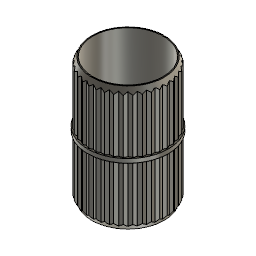
complete-v2-connector-pipe (Autodesk Fusion 360 design; units mm, degrees)
Autodesk Fusion 360 part; units mm, degrees
ref_plane "Arbeitsebene1" through (0, 0, -30) normal (0, 0, 1) x (1, 0, 0)
sketch "Skizze1" plane through (0, 0, -30) normal (0, 0, 1) x (1, 0, 0)
  circle A0 centre (0, 0) radius 17
  line L0 (19, 0) -> (18.33, 1.6037)
  line L1 (18.33, 1.6037) -> (18.7113, 3.2993)
  line L2 (18.7113, 3.2993) -> (17.773, 4.7623)
  line L3 (17.773, 4.7623) -> (17.8542, 6.4984)
  line L4 (17.8542, 6.4984) -> (16.6761, 7.7762)
  line L5 (16.6761, 7.7762) -> (16.4545, 9.5)
  line L6 (16.4545, 9.5) -> (15.0724, 10.5538)
  line L7 (15.0724, 10.5538) -> (14.5548, 12.213)
  line L8 (14.5548, 12.213) -> (13.0108, 13.0108)
  line L9 (13.0108, 13.0108) -> (12.213, 14.5548)
  line L10 (12.213, 14.5548) -> (10.5538, 15.0724)
  line L11 (10.5538, 15.0724) -> (9.5, 16.4545)
  line L12 (9.5, 16.4545) -> (7.7762, 16.6761)
  line L13 (7.7762, 16.6761) -> (6.4984, 17.8542)
  line L14 (6.4984, 17.8542) -> (4.7623, 17.773)
  line L15 (4.7623, 17.773) -> (3.2993, 18.7113)
  line L16 (3.2993, 18.7113) -> (1.6037, 18.33)
  line L17 (1.6037, 18.33) -> (0, 19)
  line L18 (0, 19) -> (-1.6037, 18.33)
  line L19 (-1.6037, 18.33) -> (-3.2993, 18.7113)
  line L20 (-3.2993, 18.7113) -> (-4.7623, 17.773)
  line L21 (-4.7623, 17.773) -> (-6.4984, 17.8542)
  line L22 (-6.4984, 17.8542) -> (-7.7762, 16.6761)
  line L23 (-7.7762, 16.6761) -> (-9.5, 16.4545)
  line L24 (-9.5, 16.4545) -> (-10.5538, 15.0724)
  line L25 (-10.5538, 15.0724) -> (-12.213, 14.5548)
  line L26 (-12.213, 14.5548) -> (-13.0108, 13.0108)
  line L27 (-13.0108, 13.0108) -> (-14.5548, 12.213)
  line L28 (-14.5548, 12.213) -> (-15.0724, 10.5538)
  line L29 (-15.0724, 10.5538) -> (-16.4545, 9.5)
  line L30 (-16.4545, 9.5) -> (-16.6761, 7.7762)
  line L31 (-16.6761, 7.7762) -> (-17.8542, 6.4984)
  line L32 (-17.8542, 6.4984) -> (-17.773, 4.7623)
  line L33 (-17.773, 4.7623) -> (-18.7113, 3.2993)
  line L34 (-18.7113, 3.2993) -> (-18.33, 1.6037)
  line L35 (-18.33, 1.6037) -> (-19, 0)
  line L36 (-19, 0) -> (-18.33, -1.6037)
  line L37 (-18.33, -1.6037) -> (-18.7113, -3.2993)
  line L38 (-18.7113, -3.2993) -> (-17.773, -4.7623)
  line L39 (-17.773, -4.7623) -> (-17.8542, -6.4984)
  line L40 (-17.8542, -6.4984) -> (-16.6761, -7.7762)
  line L41 (-16.6761, -7.7762) -> (-16.4545, -9.5)
  line L42 (-16.4545, -9.5) -> (-15.0724, -10.5538)
  line L43 (-15.0724, -10.5538) -> (-14.5548, -12.213)
  line L44 (-14.5548, -12.213) -> (-13.0108, -13.0108)
  line L45 (-13.0108, -13.0108) -> (-12.213, -14.5548)
  line L46 (-12.213, -14.5548) -> (-10.5538, -15.0724)
  line L47 (-10.5538, -15.0724) -> (-9.5, -16.4545)
  line L48 (-9.5, -16.4545) -> (-7.7762, -16.6761)
  line L49 (-7.7762, -16.6761) -> (-6.4984, -17.8542)
  line L50 (-6.4984, -17.8542) -> (-4.7623, -17.773)
  line L51 (-4.7623, -17.773) -> (-3.2993, -18.7113)
  line L52 (-3.2993, -18.7113) -> (-1.6037, -18.33)
  line L53 (-1.6037, -18.33) -> (0, -19)
  line L54 (0, -19) -> (1.6037, -18.33)
  line L55 (1.6037, -18.33) -> (3.2993, -18.7113)
  line L56 (3.2993, -18.7113) -> (4.7623, -17.773)
  line L57 (4.7623, -17.773) -> (6.4984, -17.8542)
  line L58 (6.4984, -17.8542) -> (7.7762, -16.6761)
  line L59 (7.7762, -16.6761) -> (9.5, -16.4545)
  line L60 (9.5, -16.4545) -> (10.5538, -15.0724)
  line L61 (10.5538, -15.0724) -> (12.213, -14.5548)
  line L62 (12.213, -14.5548) -> (13.0108, -13.0108)
  line L63 (13.0108, -13.0108) -> (14.5548, -12.213)
  line L64 (14.5548, -12.213) -> (15.0724, -10.5538)
  line L65 (15.0724, -10.5538) -> (16.4545, -9.5)
  line L66 (16.4545, -9.5) -> (16.6761, -7.7762)
  line L67 (16.6761, -7.7762) -> (17.8542, -6.4984)
  line L68 (17.8542, -6.4984) -> (17.773, -4.7623)
  line L69 (17.773, -4.7623) -> (18.7113, -3.2993)
  line L70 (18.7113, -3.2993) -> (18.33, -1.6037)
  line L71 (18.33, -1.6037) -> (19, 0)
extrude "Extrusion1" add sketch "Skizze1" along normal blind 60
ref_plane "Arbeitsebene2" through (0, 0, -1) normal (0, 0, 1) x (1, 0, 0)
sketch "Skizze2" plane through (0, 0, -1) normal (0, 0, 1) x (1, 0, 0)
  circle A0 centre (0, 0) radius 19.5
  circle A1 centre (0, 0) radius 17
extrude "Extrusion2" add sketch "Skizze2" along normal blind 2
sketch "Skizze3" plane through (0, 0, 0) normal (0, 1, 0) x (1, 0, 0)
  line L0 (19, -27) -> (17.5, -30)
  line L1 (17.5, -30) -> (24, -35)
  line L2 (24, -35) -> (24, -27)
  line L3 (24, -27) -> (19, -27)
revolve "Drehen1" cut sketch "Skizze3" angle 360 about axis through (0, 0, 1.75) along (0, 0, 1)
sketch "Skizze4" plane through (0, 0, 0) normal (0, 1, 0) x (1, 0, 0)
  line L0 (19, 27) -> (17.5, 30)
  line L1 (17.5, 30) -> (24, 35)
  line L2 (24, 35) -> (24, 27)
  line L3 (24, 27) -> (19, 27)
revolve "Drehen2" cut sketch "Skizze4" angle 360 about axis through (0, 0, 1.75) along (0, 0, 1)
equation "pipes_diameter = 38 mm" comment "Außendurchmesser des Verbinders an den Rippenspitzen"
equation "inner_hole_diameter = 34 mm" comment "Durchmesser der durchgehenden inneren Bohrung"
equation "connector_length = 60 mm" comment "Gesamtlänge des Verbindungsrohrs"
equation "stop_ring_width = 2 mm" comment "Breite des Anschlagrings in der Mitte (0mm = deaktiviert)"
equation "stop_ring_diameter = 39 mm" comment "Außendurchmesser des Anschlagrings in der Mitte"
equation "rib_depth = 0.6 mm" comment "Tiefe/Höhe der dreieckigen Lamellenrippen"
equation "num_ribs = 36" comment "Anzahl der umlaufenden Lamellenrippen (z. B. 36)"
equation "chamfer_size = 3 mm" comment "Größe der Einführfasen an beiden Enden (3mm)"
named bodies: "Connector_Pipe"
